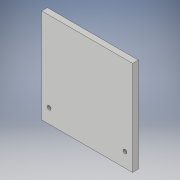
# Autodesk Inventor part: Side wall
Saved by Autodesk Inventor 2019 (Build 230136000, 136)
## iProperties
Created: 2018-08-29
Part Number: Side wall
Material: Generic
Document SubType Name: Modeling
Designer: kalakuntla1297
Density: 1 g/cm^3
Appearance: Default
Author: kalakuntla1297
Autodesk Inventor part; units mm, degrees
ref_plane "YZ Plane" through (0, 0, 0) normal (1, 0, 0) x (0, 1, 0)
ref_plane "XZ Plane" through (0, 0, 0) normal (0, 1, 0) x (-1, 0, 0)
ref_plane "XY Plane" through (0, 0, 0) normal (0, 0, 1) x (1, 0, 0)
sketch "Sketch1" plane through (0, 0, 0) normal (0, 0, 1) x (1, 0, 0)
  line L0 (0, 0) -> (200.66, 0)
  line L1 (200.66, 0) -> (200.66, 208.28)
  line L2 (200.66, 208.28) -> (0, 208.28)
  line L3 (0, 208.28) -> (0, 0)
  dimension "d0" = 200.66
  dimension "d1" = 208.28
  constraints: 8 end point, 2 parallel, 1 horizontal, 1 perpendicular
  measures "d0" distance of L0.start L0.end
  measures "d1" distance of L0.end L1.end
extrude "Extrusion1" add sketch "Sketch1" along normal blind 12.7
sketch "Sketch2" plane through (0, 0, 12.7) normal (0, 0, 1) x (1, 0, 0)
  circle A0 centre (184.023, 31.75) radius 4.1656
  line L0 (0, 0) -> (200.66, 0) projected
  line L1 (200.66, 0) -> (200.66, 208.28) projected
  circle A1 centre (16.637, 31.75) radius 4.1656
  line L2 (0, 208.28) -> (0, 0) projected
  dimension "d4" = 8.3312
  dimension "d5" = 31.75
  dimension "d6" = 16.637
  dimension "d7" = 8.3312
  dimension "d8" = 16.637
  dimension "d9" = 31.75
  constraints: 2 centre point
  measures "d4" diameter of A0
  measures "d5" distance from line of L0 A0.centre
  measures "d6" distance from line of L1 A0.centre
  measures "d7" diameter of A1
  measures "d8" distance from line of L2 A1.centre
  measures "d9" distance from line of L0 A1.centre
extrude "Extrusion2" cut sketch "Sketch2" against normal blind 25.4
body "Solid1"
